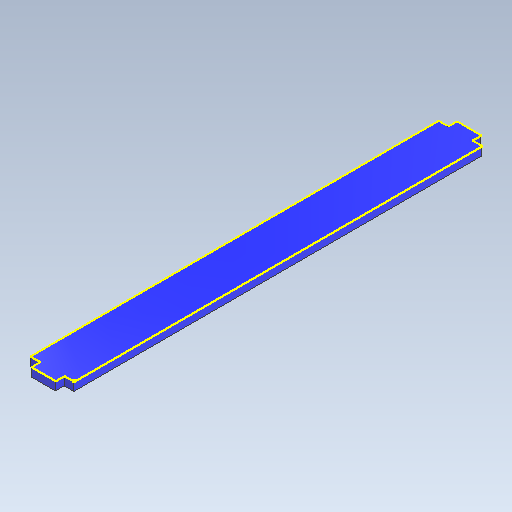
# Autodesk Inventor part: chassis_1_3
Saved by Autodesk Inventor 2022 (Build 260153000, 153)
## iProperties
Created: 2023-03-24
Part Number: chassis_1_3
Material: 一般
Document SubType Name: Modeling
Designer: Johnny Jou
Density: 79.16 g/cm^3
Appearance: 預設
Author: Johnny Jou
Autodesk Inventor part; units mm, degrees
ref_plane "YZ Plane" through (0, 0, 0) normal (1, 0, 0) x (0, 1, 0)
ref_plane "XZ Plane" through (0, 0, 0) normal (0, 1, 0) x (-1, 0, 0)
ref_plane "XY Plane" through (0, 0, 0) normal (0, 0, 1) x (1, 0, 0)
sketch "草圖1" plane through (0, 0, 0) normal (0, 1, 0) x (-1, 0, 0)
  line L0 (0, 0) -> (0, -140)
  line L1 (15, -140) -> (15, 0)
  line L2 (3.35, 0) -> (3.35, 3)
  line L3 (3.35, 3) -> (11.65, 3)
  line L4 (11.65, 3) -> (11.65, 0)
  line L5 (3.35, -140) -> (3.35, -143)
  line L6 (3.35, -143) -> (11.65, -143)
  line L7 (11.65, -143) -> (11.65, -140)
  line L8 (0, -140) -> (3.35, -140)
  line L9 (11.65, -140) -> (15, -140)
  line L10 (15, 0) -> (11.65, 0)
  line L11 (3.35, 0) -> (0, 0)
  dimension "d0" = 3
  dimension "d1" = 8.3
  dimension "d2" = 15
  dimension "d4" = 3
  dimension "d5" = 8.3
  dimension "d7" = 140
  dimension "d8" = 140
  dimension "d28" = 3.35
  dimension "d29" = 3.35
  constraints: 24 end point, 7 parallel, 4 horizontal, 2 perpendicular, 1 coincident, 1 horizontal alignment
  measures "d0" distance of L6.end L7.end
  measures "d1" distance of L5.end L6.end
  measures "d2" distance between parallel lines of L0 L1
  measures "d4" distance of L3.end L4.end
  measures "d5" distance of L2.end L3.end
  measures "d7" distance of L1.start L1.end
  measures "d8" distance of L0.start L0.end
  measures "d28" distance between parallel lines of L5 L0
  measures "d29" distance between parallel lines of L0 L2
extrude "擠出1" add sketch "草圖1" along normal blind 3
sketch "草圖3" plane through (0, 0, 0) normal (0, -1, 0) x (1, 0, 0)
  line L0 (5, 3) -> (0, 3)
  line L1 (0, 3) -> (0, -143)
  line L2 (0, -143) -> (5, -143)
  line L3 (5, -143) -> (5, 3)
  line L4 (0, 0) -> (0, -140) projected
  line L5 (-11.65, 3) -> (-3.35, 3) projected
  dimension "d24" = 146
  dimension "d25" = 5
  constraints: 8 end point, 2 collinear, 2 parallel, 1 horizontal, 1 perpendicular
  measures "d24" distance of L2.end L0.start
  measures "d25" distance between parallel lines of L1 L3
extrude "擠出3" [suppressed]
sketch "草圖2" plane through (0, 3, 0) normal (0, 1, 0) x (1, 0, 0)
  line L0 (0, 140) -> (-3.35, 140) projected
  line L1 (-3.35, 140) -> (-3.35, 143) projected
  line L2 (-3.35, 143) -> (-11.65, 143) projected
  line L3 (-11.65, 143) -> (-11.65, 140) projected
  line L4 (-11.65, 140) -> (-15, 140) projected
  line L5 (-15, 140) -> (-15, 0) projected
  line L6 (-15, 0) -> (-11.65, 0) projected
  line L7 (-11.65, 0) -> (-11.65, -3) projected
  line L8 (-11.65, -3) -> (-3.35, -3) projected
  line L9 (-3.35, -3) -> (-3.35, 0) projected
  line L10 (-3.35, 0) -> (0, 0) projected
  line L11 (-4, 134) -> (1, 134)
  line L12 (1, 134) -> (1, 6)
  line L13 (1, 6) -> (-4, 6)
  line L14 (-4, 6) -> (-4, 134)
  line L15 (-4, 67.5707) -> (-4, 72.4293)
  line L16 (-5, 72.4293) -> (-5, 67.5707)
  line L17 (5, 143) -> (5, -3) projected
  line L18 (0, 0) -> (0, 140) projected
  dimension "d17" = 5
  dimension "d19" = 6
  dimension "d20" = 6
  dimension "d30" = 4
  constraints: 12 end point, 3 parallel, 1 horizontal, 1 perpendicular, 1 point on line
  measures "d17" distance of L12.end L13.end
  measures "d19" distance between parallel lines of L10 L13
  measures "d20" distance between parallel lines of L0 L11
  measures "d30" distance between parallel lines of L17 L12
extrude "擠出2" [suppressed]
sketch "草圖4" plane through (0, 3, 0) normal (0, 1, 0) x (1, 0, 0)
  line L0 (0, 0) -> (0, 140) projected
  line L1 (0, 140) -> (-3.35, 140) projected
  line L2 (-3.35, 140) -> (-3.35, 143) projected
  line L3 (-3.35, 143) -> (-11.65, 143) projected
  line L4 (-11.65, 143) -> (-11.65, 140) projected
  line L5 (-11.65, 140) -> (-15, 140) projected
  line L6 (-15, 140) -> (-15, 0) projected
  line L7 (-15, 0) -> (-11.65, 0) projected
  line L8 (-11.65, 0) -> (-11.65, -3) projected
  line L9 (-11.65, -3) -> (-3.35, -3) projected
  line L10 (-3.35, -3) -> (-3.35, 0) projected
  line L11 (-3.35, 0) -> (0, 0) projected
equation "\"d29\" = d28"
